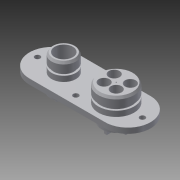
# Autodesk Inventor part: Connector
Saved by Autodesk Inventor 2014 SP2 (Build 180246200, 246)
## iProperties
Created: 2015-09-17
Part Number: Connector
Material: ABS Plastic
Document SubType Name: Modeling
Designer: Lukasz Szmit
Density: 1.06 g/cm^3
Appearance: Smooth - White
Mass: 22.7046 g
Surface Area: 127.542 cm^2
Volume: 21.4194 cm^3
Author: Lukasz Szmit
Autodesk Inventor part; units mm, degrees
sketch "Slot" plane through (0, 0, 0) normal (0, 0, 1) x (1, 0, 0)
  line L0 (-28.1189, 16.8852) -> (28.1311, 16.8648)
  line L1 (44.9939, -0.0102) -> (44.9939, -0.0102)
  line L2 (27.4299, -16.8586) -> (-27.6697, -16.8586)
  line L3 (-45, 0.0102) -> (-45, 0.0102)
  arc A0 (-28.1189, 16.8852) -> (-27.6697, -16.8586) centre (-28.125, 0.0102) ccw
  arc A1 (27.4299, -16.8586) -> (28.1311, 16.8648) centre (28.125, -0.0041) ccw
  point P0 (0, 0)
  point P1 (-45, 16.8914)
  point P2 (45, 16.8586)
  point P3 (-45, -16.8586)
  dimension "d7" = 4
  dimension "d8" = 4
  dimension "d9" = 4
  dimension "d10" = 4
  dimension "d11" = 78
  dimension "d16" = 21
  dimension "d17" = 39
  dimension "d0" = 90
  dimension "d1" = 33.75
  dimension "d2" = 16.875
  dimension "d4" = 16.875
  dimension "d6" = 90
  dimension "d19" = 56.25
  dimension "d20" = 28.125
  constraints: 8 end point, 8 point on circle, 6 point on line, 4 tangent, 2 centre point, 2 perpendicular
  measures "d0" distance of point (-45, 16.891) point (45, 16.859)
  measures "d1" distance of point (-45, -16.859) point (-45, 16.891)
  measures "d2" distance from line of point (0, 0) L0
  measures "d4" radius of A0
  measures "d6" horizontal distance of point (45, 16.859) point (-45, -16.859)
  measures "d19" distance of A1.centre A0.centre
  measures "d20" distance of point (0, 0) A0.centre
sketch "Holes" plane through (0, 0, 0) normal (0, 0, 1) x (1, 0, 0)
  circle A0 centre (-39, 0) radius 2
  circle A1 centre (39, 0) radius 2
  circle A2 centre (0, -10.5) radius 2
  circle A3 centre (0, 10.5) radius 2
  point P0 (0, 0)
  point P1 (-3.3578, 23.5)
  dimension "d7" = 4
  dimension "d8" = 4
  dimension "d9" = 4
  dimension "d10" = 4
  dimension "d11" = 78
  dimension "d16" = 21
  dimension "d17" = 39
  constraints: 4 centre point
  measures "d7" diameter of A0
  measures "d8" diameter of A2
  measures "d9" diameter of A1
  measures "d10" diameter of A3
  measures "d11" distance of A1.centre A0.centre
  measures "d16" distance of A3.centre A2.centre
  measures "d17" horizontal distance of A1.centre A2.centre
extrude "Extrusion1" add sketch "Slot" against normal blind 4
hole "Hole1" at (0, 10.5, 0) at (39, 0, 0) at (0, -10.5, 0) at (-39, 0, 0) direction (0, 0, -1) diameter 4 end through all
ref_plane "Work Plane1" through (0, 0, 13) normal (0, 0, 1) x (1, 0, 0)
sketch "Socket Outline" plane through (0, 0, 13) normal (0, 0, 1) x (1, 0, 0)
  line L0 (-19.5, 12) -> (19.5, 12) construction
  line L1 (31.5, 0) -> (31.5, 0) construction
  line L2 (19.5, -12) -> (-19.5, -12) construction
  line L3 (-31.5, 0) -> (-31.5, 0) construction
  arc A0 (-19.5, 12) -> (-19.5, -12) centre (-19.5, 0) ccw construction
  arc A1 (19.5, -12) -> (19.5, 12) centre (19.5, 0) ccw construction
  point P0 (0, 0)
  point P1 (-31.5, 12)
  point P2 (31.5, 12)
  point P3 (-31.5, -12)
  dimension "d31" = 63
  dimension "d32" = 24
  dimension "d33" = 12
  dimension "d34" = 12
  dimension "d35" = 63
  dimension "d36" = 39
  dimension "d37" = 19.5
  constraints: 8 end point, 8 point on circle, 6 point on line, 4 tangent, 2 centre point, 2 perpendicular, 1 parallel
  measures "d31" distance of point (-31.5, 12) point (31.5, 12)
  measures "d32" distance of point (-31.5, -12) point (-31.5, 12)
  measures "d33" distance from line of point (0, 0) L0
  measures "d34" radius of A0
  measures "d35" horizontal distance of point (31.5, 12) point (-31.5, -12)
  measures "d36" distance of A1.centre A0.centre
  measures "d37" distance of point (0, 0) A0.centre
sketch "Small Socket" plane through (0, 0, 13) normal (0, 0, 1) x (1, 0, 0)
  circle A0 centre (-19.5, 0) radius 0.0027
  circle A1 centre (-19.5, 0) radius 9
  circle A2 centre (-39, 0) radius 2 projected
  point P0 (0, 0)
  dimension "d38" = 18
  dimension "d40" = 19.5
  dimension "d43" = 19.5
  constraints: 2 centre point, 1 coincident
  measures "d38" diameter of A1
  measures "d40" distance of A1.centre A2.centre
  measures "d43" distance of point (0, 0) A0.centre
sketch "Big Socket" plane through (0, 0, 13) normal (0, 0, 1) x (1, 0, 0)
  circle A0 centre (19.5, 0) radius 13.25
  circle A1 centre (39, 0) radius 2 projected
  point P0 (0, 0)
  dimension "d39" = 26.5
  dimension "d41" = 19.5
  dimension "d42" = 19.5
  constraints: 1 centre point
  measures "d39" diameter of A0
  measures "d41" distance of A1.centre A0.centre
  measures "d42" distance of point (0, 0) A0.centre
extrude "Extrusion2" add sketch "Small Socket" against normal blind 13 contours A1
extrude "Extrusion3" add sketch "Big Socket" against normal blind 13 contours A0
ref_plane "Work Plane3" through (-19.5, 0, 13) normal (1, 0, 0) x (0, 1, 0)
sketch "Sketch7" plane through (-19.5, 0, 13) normal (1, 0, 0) x (0, 1, 0)
  line L0 (-9, -13) -> (-9, 0) construction
  line L1 (-9, 0) -> (-0.0027, 0) construction
  line L2 (-0.0027, 0) -> (-0.0027, -13) construction
  line L3 (-0.0027, -13) -> (0.0027, -13) construction
  line L4 (0.0027, -13) -> (0.0027, 0) construction
  line L5 (0.0027, 0) -> (9, 0) construction
  line L6 (9, 0) -> (9, -13) construction
  line L7 (9, -13) -> (16.8821, -13) construction
  line L8 (16.8821, -13) -> (16.8821, -17) construction
  line L9 (16.8821, -17) -> (-16.8586, -17) construction
  line L10 (-16.8586, -17) -> (-16.8586, -13) construction
  line L11 (-16.8586, -13) -> (-9, -13) construction
  line L12 (9, -7.1) -> (7.5, -7.1)
  line L13 (7.5, -7.1) -> (7.5, -9)
  line L14 (7.5, -9) -> (9, -9)
  line L15 (9, -9) -> (9, -7.1)
  line L16 (0, 3.4) -> (0, -20.4) projected
  point P0 (0, -13)
  dimension "d53" = 1.5
  dimension "d54" = 1.9
  dimension "d55" = 4
  constraints: 8 end point, 1 perpendicular, 1 point on line
  measures "d53" distance of L12.start L12.end
  measures "d54" distance of L12.end L13.end
  measures "d55" distance between parallel lines of L7 L14
revolve "Revolution2" cut sketch "Sketch7" angle 360 about axis through (-19.5, 0, 13) along (0, 0, -1)
ref_plane "Work Plane4" through (19.5, 0, 13) normal (1, 0, 0) x (0, 1, 0)
sketch "Sketch8" plane through (19.5, 0, 13) normal (1, 0, 0) x (0, 1, 0)
  line L0 (-13.25, -13) -> (-13.25, 0) construction
  line L1 (-13.25, 0) -> (13.25, 0) construction
  line L2 (13.25, 0) -> (13.25, -13) construction
  line L3 (13.25, -13) -> (16.8679, -13) construction
  line L4 (16.8679, -13) -> (16.8679, -17) construction
  line L5 (16.8679, -17) -> (-16.8586, -17) construction
  line L6 (-16.8586, -17) -> (-16.8586, -13) construction
  line L7 (-16.8586, -13) -> (-13.25, -13) construction
  line L8 (-13.25, -7.1) -> (-11.75, -7.1)
  line L9 (-11.75, -7.1) -> (-11.75, -9)
  line L10 (-11.75, -9) -> (-13.25, -9)
  line L11 (-13.25, -9) -> (-13.25, -7.1)
  line L12 (0, 3.4) -> (0, -20.4) projected
  point P0 (0, -13)
  dimension "d57" = 1.5
  dimension "d58" = 1.9
  dimension "d59" = 4
  constraints: 8 end point, 2 perpendicular, 1 parallel, 1 point on line
  measures "d57" distance of L8.start L8.end
  measures "d58" distance of L8.end L9.end
  measures "d59" distance from line of L0.start L10
revolve "Revolution3" cut sketch "Sketch8" angle 360 about axis through (19.5, 0, 13) along (0, 0, -1)
ref_plane "Work Plane5" through (0, 0, 13) normal (0, 0, 1) x (1, 0, 0)
sketch "Sketch9" plane through (19.5, 0, 13) normal (0, 0, 1) x (1, 0, 0)
  circle A0 centre (0, 0) radius 13.25 construction
  circle A1 centre (-6, 4.5) radius 4
  circle A2 centre (6, 4.5) radius 4
  circle A3 centre (-4.5, -4.5) radius 4
  circle A4 centre (4.5, -4.5) radius 4
  point P0 (-19.5, 0)
  dimension "d62" = 8
  dimension "d63" = 6
  dimension "d64" = 4.5
  dimension "d65" = 4.5
  dimension "d66" = 4.5
  dimension "d67" = 4.5
  dimension "d68" = 6
  dimension "d69" = 8
  dimension "d70" = 8
  dimension "d71" = 8
  dimension "d72" = 4.5
  dimension "d73" = 4.5
  constraints: 4 centre point
  measures "d62" diameter of A1
  measures "d63" horizontal distance of A0.centre A1.centre
  measures "d64" vertical distance of A0.centre A1.centre
  measures "d65" horizontal distance of A3.centre A0.centre
  measures "d66" vertical distance of A0.centre A2.centre
  measures "d67" horizontal distance of A0.centre A4.centre
  measures "d68" horizontal distance of A0.centre A2.centre
  measures "d69" diameter of A2
  measures "d70" diameter of A3
  measures "d71" diameter of A4
  measures "d72" horizontal distance of A0.centre A3.centre
  measures "d73" horizontal distance of A4.centre A0.centre
hole "Hole2" at (24, -4.5, 13) at (15, -4.5, 13) at (13.5, 4.5, 13) at (25.5, 4.5, 13) direction (0, 0, -1) diameter 8 depth 13.5
sketch "Sketch10" plane through (19.5, 0, 13) normal (0, 0, 1) x (1, 0, 0)
  circle A0 centre (0, 0) radius 13.25 projected
  circle A1 centre (0, 0) radius 0.375
  point P0 (-19.5, 0)
  dimension "d88" = 0.75
  constraints: 1 centre point, 1 coincident
  measures "d88" diameter of A1
hole "Hole3" at (19.5, 0, 13) direction (0, 0, -1) diameter 0.75 depth 37.75
sketch "Sketch11" plane through (-19.5, 0, 13) normal (0, 0, 1) x (1, 0, 0)
  circle A0 centre (0, 0) radius 9 projected
  point P0 (19.5, 0)
  constraints: 1 coincident
hole "Hole4" at (-19.5, 0, 13) direction (0, 0, -1) diameter 13.5 depth 13.5
chamfer "Chamfer1" distance 1 angle 60 1 edges at (6.25, 0, 13) measured on face at (20.0324, 8.8993, 13)
chamfer "Chamfer2" distance 1 angle 60 1 edges at (-28.5, 0, 13) measured on face at (-11.3536, -0.9892, 13)
sketch "Sketch15" plane through (0, 0, -4) normal (0, 0, -1) x (-1, 0, 0)
  circle A0 centre (-19.5, 0) radius 0.375 projected
  circle A1 centre (-19.5, 0) radius 10.75
  circle A2 centre (19.5, 0) radius 9.825
  circle A3 centre (-19.5, 0) radius 0.375 projected
  circle A4 centre (-19.5, 0) radius 13.25 projected
  point P0 (0, 0)
  dimension "d122" = 21.5
  dimension "d123" = 19.65
  dimension "d124" = 39
  constraints: 2 centre point, 1 coincident, 1 concentric
  measures "d122" diameter of A1
  measures "d123" diameter of A2
  measures "d124" distance of A2.centre A1.centre
extrude "Extrusion4" add sketch "Sketch15" along normal blind 8 contours A1 | A2
sketch "Sketch38" plane through (13.5, 4.5, -0.5) normal (0, 0, 1) x (1, 0, 0)
  circle A0 centre (6, -4.5) radius 0.375 construction
  circle A1 centre (0, 0) radius 4 construction
  circle A2 centre (10.5, -9) radius 4 construction
  circle A3 centre (1.5, -9) radius 4 construction
  circle A4 centre (12, 0) radius 4 construction
  circle A5 centre (-13.5, -15) radius 2 construction
  circle A6 centre (-13.5, 6) radius 2 construction
  circle A7 centre (25.5, -4.5) radius 2 construction
  circle A8 centre (-52.5, -4.5) radius 2 construction
  line L0 (13.9299, -21.3586) -> (-41.1698, -21.3586) construction
  arc A9 (-41.6189, 12.3852) -> (-41.1698, -21.3586) centre (-41.625, -4.4898) ccw construction
  line L1 (-41.6189, 12.3852) -> (14.6311, 12.3648) construction
  arc A10 (13.9299, -21.3586) -> (14.6311, 12.3648) centre (14.625, -4.5041) ccw construction
  circle A11 centre (-33, -4.5) radius 6.75 projected
  point P0 (-13.5, -4.5)
  constraints: 4 coincident
hole "Hole14" at (13.5, 4.5, -0.5) at (25.5, 4.5, -0.5) at (24, -4.5, -0.5) at (15, -4.5, -0.5) at (-19.5, 0, -0.5) direction (0, 0, -1) diameter 6 depth 1
sketch "Sketch39" plane through (24, -4.5, -1.5) normal (0, 0, 1) x (1, 0, 0)
  circle A0 centre (-9, 0) radius 3 construction
  circle A1 centre (1.5, 9) radius 3 construction
  circle A2 centre (-10.5, 9) radius 3 construction
  circle A3 centre (0, 0) radius 3 construction
  circle A4 centre (-43.5, 4.5) radius 3 construction
  circle A5 centre (-4.5, 4.5) radius 0.375 construction
  circle A6 centre (-24, -6) radius 2 construction
  circle A7 centre (-24, 15) radius 2 construction
  circle A8 centre (15, 4.5) radius 2 construction
  circle A9 centre (-63, 4.5) radius 2 construction
  line L0 (3.4299, -12.3586) -> (-51.6698, -12.3586) construction
  arc A10 (-52.1189, 21.3852) -> (-51.6698, -12.3586) centre (-52.125, 4.5102) ccw construction
  line L1 (-52.1189, 21.3852) -> (4.1311, 21.3648) construction
  arc A11 (3.4299, -12.3586) -> (4.1311, 21.3648) centre (4.125, 4.4959) ccw construction
  point P0 (-24, 4.5)
  constraints: 5 coincident
hole "Hole15" at (13.5, 4.5, -1.5) at (25.5, 4.5, -1.5) at (24, -4.5, -1.5) at (15, -4.5, -1.5) at (-19.5, 0, -1.5) direction (0, 0, -1) diameter 3 end through all
sketch "Sketch40" plane through (19.5, 0, -12) normal (0, 0, -1) x (-1, 0, 0)
  circle A0 centre (0, 0) radius 0.375 construction
  circle A1 centre (4.5, -4.5) radius 1.5 construction
  circle A2 centre (-6, 4.5) radius 1.5 construction
  circle A3 centre (6, 4.5) radius 1.5 construction
  circle A4 centre (-4.5, -4.5) radius 1.5 construction
  circle A5 centre (39, 0) radius 1.5 construction
  circle A6 centre (0, 0) radius 10.75 construction
  circle A7 centre (39, 0) radius 9.825 construction
  circle A8 centre (0, 0) radius 0.375 construction
  line L0 (1, 8) -> (1, 6)
  line L1 (6, 1) -> (8, 1)
  line L2 (8, 1) -> (8, -1)
  line L3 (8, -1) -> (3, -1)
  line L4 (1, -3) -> (1, -8)
  line L5 (1, -8) -> (-1, -8)
  line L6 (-1, -8) -> (-1, -3)
  line L7 (-3, -1) -> (-8, -1)
  line L8 (-8, -1) -> (-8, 1)
  line L9 (-8, 1) -> (-6, 1)
  line L10 (-1, 6) -> (-1, 8)
  line L11 (-1, 8) -> (1, 8)
  arc A9 (-6, 1) -> (-1, 6) centre (-6, 6) ccw
  arc A10 (1, 6) -> (6, 1) centre (6, 6) ccw
  arc A11 (-1, -3) -> (-3, -1) centre (-3, -3) ccw
  arc A12 (3, -1) -> (1, -3) centre (3, -3) ccw
  point P0 (19.5, 0)
  point P1 (1, 1)
  point P2 (1, -1)
  point P3 (-1, -1)
  dimension "d357" = 2
  dimension "d358" = 2
  dimension "d359" = 2
  dimension "d360" = 2
  dimension "d361" = 7
  dimension "d362" = 7
  dimension "d363" = 7
  dimension "d366" = 8
  dimension "d367" = 8
  dimension "d368" = 5
  dimension "d369" = 2
  constraints: 24 end point, 8 point on circle, 8 tangent, 6 point on line, 4 centre point, 4 collinear, 4 perpendicular, 2 equal radius
  measures "d357" distance of L10.end L0.start
  measures "d358" distance of L1.end L2.end
  measures "d359" distance of L7.end L8.end
  measures "d360" distance of L4.end L5.end
  measures "d361" distance of L0.start point (1, 1)
  measures "d362" distance of point (1, -1) L4.end
  measures "d363" distance of point (-1, -1) L7.end
  measures "d366" distance from line of L11 A0.centre
  measures "d367" distance from line of A0.centre L2
  measures "d368" radius of A9
  measures "d369" radius of A11
extrude "Extrusion6" add sketch "Sketch40" along normal blind 4.5
sketch "Sketch41" plane through (19.5, 0, -16.5) normal (0, 0, -1) x (-1, 0, 0)
  point P0 (19.5, 0)
  point P1 (0, 0)
hole "Hole16" at (19.5, 0, -16.5) direction (0, 0, 1) diameter 0.75 end through all
sketch "Sketch42" plane through (-19.5, 0, -12) normal (0, 0, -1) x (-1, 0, 0)
  arc A0 (-38, 6) -> (-33, 1) centre (-33, 6) ccw construction
  line L0 (-33, 1) -> (-31, 1) construction
  line L1 (-31, 1) -> (-31, -1) construction
  line L2 (-31, -1) -> (-36, -1) construction
  arc A1 (-36, -1) -> (-38, -3) centre (-36, -3) ccw construction
  line L3 (-38, -3) -> (-38, -8) construction
  line L4 (-38, -8) -> (-40, -8) construction
  line L5 (-40, -8) -> (-40, -3) construction
  arc A2 (-40, -3) -> (-42, -1) centre (-42, -3) ccw construction
  line L6 (-42, -1) -> (-47, -1) construction
  line L7 (-47, -1) -> (-47, 1) construction
  line L8 (-47, 1) -> (-45, 1) construction
  arc A3 (-45, 1) -> (-40, 6) centre (-45, 6) ccw construction
  line L9 (-40, 6) -> (-40, 8) construction
  line L10 (-40, 8) -> (-38, 8) construction
  line L11 (-38, 8) -> (-38, 6) construction
  circle A4 centre (-34.5, -4.5) radius 1.5 construction
  circle A5 centre (-45, 4.5) radius 1.5 construction
  circle A6 centre (-33, 4.5) radius 1.5 construction
  circle A7 centre (-43.5, -4.5) radius 1.5 construction
  circle A8 centre (0, 0) radius 1.5 construction
  circle A9 centre (-39, 0) radius 10.75 construction
  circle A10 centre (0, 0) radius 9.825 construction
  circle A11 centre (-39, 0) radius 0.375 construction
  arc A12 (2.25, -3.8971) -> (0, 4.5) centre (0, 0) ccw
  arc A13 (0, -3.75) -> (0, 3.75) centre (0, 0) ccw
  arc A14 (0, -5.5) -> (2.75, -4.7631) centre (0, 0) ccw
  line L12 (2.25, -3.8971) -> (2.75, -4.7631)
  line L13 (0, 4.5) -> (0, 3.75)
  line L14 (0, -3.75) -> (0, -5.5)
  point P0 (-19.5, 0)
  dimension "d379" = 9
  dimension "d380" = 7.5
  dimension "d381" = 11
  constraints: 6 end point, 6 point on circle, 3 centre point, 1 coincident
  measures "d379" diameter of A12
  measures "d380" diameter of A13
  measures "d381" diameter of A14
extrude "Extrusion7" add sketch "Sketch42" along normal blind 4.5
sketch "Sketch43" plane through (-19.5, 0, -16.5) normal (0, 0, -1) x (-1, 0, 0)
  arc A0 (2.25, -3.8971) -> (0, 4.5) centre (0, 0) ccw construction
  line L0 (2.25, -3.8971) -> (2.75, -4.7631) construction
  arc A1 (0, -5.5) -> (2.75, -4.7631) centre (0, 0) ccw construction
  line L1 (0, -5.5) -> (0, -3.75) construction
  arc A2 (0, -3.75) -> (0, 3.75) centre (0, 0) ccw construction
  line L2 (0, 3.75) -> (0, 4.5) construction
  arc A3 (2.25, -3.8971) -> (0, 4.5) centre (0, 0) ccw construction
  arc A4 (-38, 6) -> (-33, 1) centre (-33, 6) ccw construction
  line L3 (-33, 1) -> (-31, 1) construction
  line L4 (-31, 1) -> (-31, -1) construction
  line L5 (-31, -1) -> (-36, -1) construction
  arc A5 (-36, -1) -> (-38, -3) centre (-36, -3) ccw construction
  line L6 (-38, -3) -> (-38, -8) construction
  line L7 (-38, -8) -> (-40, -8) construction
  line L8 (-40, -8) -> (-40, -3) construction
  arc A6 (-40, -3) -> (-42, -1) centre (-42, -3) ccw construction
  line L9 (-42, -1) -> (-47, -1) construction
  line L10 (-47, -1) -> (-47, 1) construction
  line L11 (-47, 1) -> (-45, 1) construction
  arc A7 (-45, 1) -> (-40, 6) centre (-45, 6) ccw construction
  line L12 (-40, 6) -> (-40, 8) construction
  line L13 (-40, 8) -> (-38, 8) construction
  line L14 (-38, 8) -> (-38, 6) construction
  circle A8 centre (-39, 0) radius 0.375 construction
  point P0 (-19.5, 0)
  point P1 (1.0684, -4.25)
  dimension "d385" = 4.25
  measures "d385" vertical distance of point (1.068, -4.25) A0.centre
hole "Hole17" at (-20.5684, -4.25, -16.5) direction (0, 0, 1) diameter 0.75 end through all
sketch "Sketch44" plane through (-19.5, 0, -0.5) normal (0, 0, 1) x (1, 0, 0)
  arc A0 (-5.1199, 2.6171) -> (-5.1123, -2.6318) centre (0, 0) ccw
  arc A1 (-5.9841, 3.123) -> (-5.982, -3.127) centre (0, 0) ccw
  line L0 (-5.1123, -2.6318) -> (-5.982, -3.127)
  line L1 (-5.1199, 2.6171) -> (-5.9841, 3.123)
  circle A2 centre (0, 0) radius 3 projected
  point P0 (19.5, 0)
  dimension "d393" = 11.5
  dimension "d394" = 13.5
  dimension "d401" = 1
  dimension "d402" = 60
  constraints: 4 end point, 4 point on circle, 2 centre point, 1 concentric
  measures "d393" diameter of A0
  measures "d394" diameter of A1
  measures "d401" radial gap between concentric circles of A1 A0
  measures "d402" angle of L0 L1
extrude "Extrusion8" cut sketch "Sketch44" against normal through all contours A0 L0 A1 L1
equation "\"d8\" = d7"
equation "\"d9\" = d7"
equation "\"d10\" = d7"
equation "\"d2\" = 0.5 * d1"
equation "\"d4\" = 0.5 * d1"
equation "\"d6\" = d0"
equation "\"d19\" = d0 - 2 * d4"
equation "\"d20\" = 0.5 * d19"
equation "\"d33\" = 0.5 * d32"
equation "\"d34\" = 0.5 * d32"
equation "\"d35\" = d31"
equation "\"d36\" = d31 - 2 * d34"
equation "\"d37\" = 0.5 * d36"
equation "\"d40\" = d41"
equation "\"d43\" = d41"
equation "\"d42\" = d41"
equation "\"d54\" = d58"
equation "\"d65\" = d64"
equation "\"d66\" = d64"
equation "\"d67\" = d64"
equation "\"d68\" = d63"
equation "\"d69\" = d62"
equation "\"d70\" = d62"
equation "\"d71\" = d62"
equation "\"d73\" = d72"
body "Solid1"
